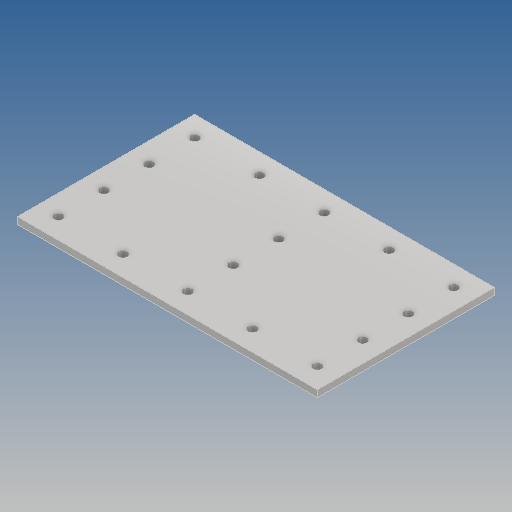
# Autodesk Inventor part: 100-10-FRAME-DIFFERENTIAL-REINF-01
Saved by Autodesk Inventor 2018.2 (Build 222227000, 227)
## iProperties
Manager: feesmrt
Company: FRANCOR
Part Number: 100-10-FRAME-DIFFERENTIAL-REINF-01
Project: Rescue Robot
Cost Center: -
Material: Aluminium 6061
Document SubType Name: Modeling
Designer: feesmrt
Engineer: feesmrt
Authority: feesmrt
Density: 2.7 g/cm^3
Appearance: Aluminium - dunkel
Description: Differentialaufnahme Verstärkung
Stock Number: 100-10-FRAME-DIFFERENTIAL-REINF-01
Subject: Rescue Robot
Author: feesmrt
Revision Number: 1
Title: Differentialaufnahme Verstärkung
Autodesk Inventor part; units mm, degrees
ref_plane "YZ Plane" through (0, 0, 0) normal (1, 0, 0) x (0, 1, 0)
ref_plane "XZ Plane" through (0, 0, 0) normal (0, 1, 0) x (-1, 0, 0)
ref_plane "XY Plane" through (0, 0, 0) normal (0, 0, 1) x (1, 0, 0)
sketch "Skizze1" plane through (0, 0, 0) normal (0, 0, 1) x (1, 0, 0)
  line L0 (-110, -65) -> (110, -65)
  line L1 (110, -65) -> (110, 65)
  line L2 (110, 65) -> (-110, 65)
  line L3 (-110, 65) -> (-110, -65)
  line L4 (-110, -65) -> (110, 65) construction
  line L5 (110, -65) -> (-110, 65) construction
  point P0 (0, 0)
  dimension "d0" = 220
  dimension "d1" = 130
  constraints: 12 end point, 2 midpoint, 2 parallel, 1 horizontal, 1 perpendicular
  measures "d0" distance of L1.end L2.end
  measures "d1" distance of L0.end L1.end
extrude "Grundkörper" add sketch "Skizze1" along normal blind 5
sketch "Skizze2" plane through (0, 0, 5) normal (0, 0, 1) x (1, 0, 0)
  line L0 (110, 65) -> (-110, 65) construction
  line L1 (-110, 65) -> (-110, -65) construction
  line L2 (110, -65) -> (110, 65) construction
  line L3 (-110, -65) -> (110, -65) construction
  line L4 (-95, -50) -> (95, -50) construction
  line L5 (95, -50) -> (95, 50) construction
  line L6 (95, 50) -> (-95, 50) construction
  line L7 (-95, 50) -> (-95, -50) construction
  line L8 (-95, -50) -> (95, 50) construction
  line L9 (95, -50) -> (-95, 50) construction
  line L10 (0, 65) -> (0, -65) construction
  point P0 (0, 0)
  point P1 (0, 50)
  point P2 (-95, 16.6667)
  point P3 (-95, -16.6667)
  point P4 (-95, -50)
  point P5 (0, 50)
  point P6 (0, 16.6667)
  point P7 (0, -16.6667)
  point P8 (0, -50)
  point P9 (-47.5, 50)
  point P10 (-47.5, -50)
  point P11 (0, 50)
  point P12 (0, -50)
  point P13 (95, 50)
  point P14 (95, 16.6667)
  point P15 (95, -16.6667)
  point P16 (95, -50)
  point P17 (95, -50)
  point P18 (47.5, 50)
  point P19 (47.5, -50)
  dimension "d4" = 15
  dimension "d5" = 15
  dimension "d6" = 100
  dimension "d7" = 190
  dimension "d17" = 33.3333
  dimension "d20" = 95
  dimension "d25" = 47.5
  constraints: 14 end point, 7 symmetric about line, 5 midpoint, 3 horizontal, 2 parallel, 2 point on line, 2 vertical alignment, 1 coincident, 1 perpendicular, 1 vertical, 11 other
  measures "d4" distance between parallel lines of L0 L6
  measures "d5" distance between parallel lines of L2 L5
  measures "d6" distance of L6.end L4.start
  measures "d7" distance of L5.end L6.end
  measures "d17" distance of point (-95, 50) point (-95, 16.667)
  measures "d20" distance of point (-95, 50) point (0, 50)
  measures "d25" distance of point (-95, 50) point (-47.5, 50)
hole "Boh_M6" at (-95, 50, 5) at (0, 50, 5) at (-95, 16.6667, 5) at (-95, -16.6667, 5) at (-95, -50, 5) at (-95, -50, 5) at (0, 16.6667, 5) at (0, -16.6667, 5) at (0, -50, 5) at (-47.5, 50, 5) at (-47.5, -50, 5) at (47.5, 50, 5) at (95, 50, 5) at (95, 16.6667, 5) at (95, -16.6667, 5) at (95, -50, 5) at (95, -50, 5) at (47.5, -50, 5) direction (0, 0, -1) diameter 6.6 end through all
equation "\"d0\" = Chassis_Width"
equation "\"d17\" = 0.333333 * d6"
equation "\"d20\" = 0.5 * d7"
equation "\"d25\" = 0.25 * d7"
equation "\"Chassis_Width\" = 220"
equation "\"Rocker_Screw_Distance\" = 32.5"
equation "\"Rocker_Screw_Distance_Bottom\" = 76"
